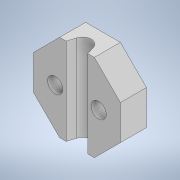
# Autodesk Inventor part: ワイヤジンバル3
Saved by Autodesk Inventor 2020 (Build 240168000, 168)
## iProperties
Created: 2019-10-22
Part Number: ワイヤジンバル3
Material: 一般
Document SubType Name: Modeling
Designer: highs
Density: 1 g/cm^3
Appearance: 既定
Author: highs
## iProperties of the stored document _3D プリント.ipt
Created: 2019-10-23
Part Number: _3D プリント
Material: 一般
Document SubType Name: Modeling
Designer: highs
Density: 1 g/cm^3
Appearance: 既定
Author: highs
Autodesk Inventor part; units mm, degrees
ref_plane "YZ Plane" through (0, 0, 0) normal (1, 0, 0) x (0, 1, 0)
ref_plane "XZ Plane" through (0, 0, 0) normal (0, 1, 0) x (-1, 0, 0)
ref_plane "XY Plane" through (0, 0, 0) normal (0, 0, 1) x (1, 0, 0)
sketch "スケッチ1" plane through (0, 0, 0) normal (0, 0, 1) x (1, 0, 0)
  line L0 (0, 0) -> (20, 0)
  line L1 (20, 0) -> (20, 20)
  line L2 (20, 20) -> (0, 20)
  line L3 (0, 20) -> (0, 0)
  line L4 (0, 10) -> (20, 10) construction
  circle A0 centre (5, 10) radius 1.75
  line L5 (10, 20) -> (10, 0) construction
  circle A1 centre (15, 10) radius 1.75
  dimension "d0" = 20
  dimension "d1" = 20
  dimension "d2" = 10
  dimension "d3" = 3.5
  dimension "d4" = 10
  constraints: 12 end point, 4 midpoint, 2 centre point, 2 horizontal, 2 parallel, 1 perpendicular, 1 point on line, 1 symmetric about line, 1 other
  measures "d0" distance of L2.end L0.start
  measures "d1" distance of L0.start L0.end
  measures "d2" distance of A1.centre A0.centre
  measures "d3" diameter of A0
  measures "d4" distance between parallel lines of L0 L4
extrude "押し出し1" add sketch "スケッチ1" along normal blind 6
sketch "スケッチ2" plane through (0, 0, 0) normal (0, -1, 0) x (1, 0, 0)
  line L0 (0, 0) -> (20, 0) construction
  line L1 (10, 0) -> (10, 6) construction
  line L2 (0, 6) -> (20, 6) construction
  line L3 (7.5, 6) -> (8.091, 4.1087)
  line L4 (11.909, 4.1087) -> (12.5, 6)
  line L5 (7.5, 6) -> (12.5, 6)
  arc A0 (8.091, 4.1087) -> (11.909, 4.1087) centre (10, 4.7052) ccw
  point P0 (10, -2)
  dimension "d11" = 2
  dimension "d18" = 5
  dimension "d19" = 8
  constraints: 8 end point, 5 point on line, 2 midpoint, 2 point on circle, 2 tangent, 1 centre point, 1 collinear, 1 other
  measures "d11" radius of A0
  measures "d18" distance of L3.start L4.end
  measures "d19" distance from line of L2 point (10, -2)
extrude "押し出し2" cut sketch "スケッチ2" against normal through all
chamfer "面取り1" distance 6 angle 45 4 edges at (20, 20, 3) (0, 20, 3) (20, 0, 3) (0, 0, 3)
